Autodesk Inventor part; units mm, degrees
(part 2 of 2)
sketch "Sketch9" plane through (0, 0, 5.08) normal (0, 0, 1) x (1, 0, 0)
  line L0 (165.1, 177.8) -> (175.26, 177.8)
  line L1 (175.26, 177.8) -> (175.26, 172.72)
  line L2 (175.26, 172.72) -> (165.1, 172.72)
  line L3 (165.1, 172.72) -> (165.1, 177.8)
  arc A0 (32.5266, 197.2829) -> (35.5167, 193.04) centre (35.5167, 196.215) ccw projected
  line L4 (32.5266, 197.2829) -> (95.435, 373.4262) projected
  arc A1 (101.6, 372.3583) -> (95.435, 373.4262) centre (98.425, 372.3583) ccw projected
  line L5 (101.6, 372.3583) -> (101.6, 196.215) projected
  arc A2 (98.425, 193.04) -> (101.6, 196.215) centre (98.425, 196.215) ccw projected
  line L6 (98.425, 193.04) -> (35.5167, 193.04) projected
  arc A3 (188.0033, 193.04) -> (190.9934, 197.2829) centre (188.0033, 196.215) ccw projected
  line L7 (188.0033, 193.04) -> (125.095, 193.04) projected
  arc A4 (121.92, 196.215) -> (125.095, 193.04) centre (125.095, 196.215) ccw projected
  line L8 (121.92, 196.215) -> (121.92, 372.3583) projected
  arc A5 (128.085, 373.4262) -> (121.92, 372.3583) centre (125.095, 372.3583) ccw projected
  line L9 (128.085, 373.4262) -> (190.9934, 197.2829) projected
  arc A6 (29.025, 513.5979) -> (22.86, 512.53) centre (26.035, 512.53) ccw projected
  line L10 (29.025, 513.5979) -> (76.0908, 381.8139) projected
  arc A7 (76.0908, 379.6781) -> (76.0908, 381.8139) centre (73.1007, 380.746) ccw projected
  line L11 (76.0908, 379.6781) -> (29.025, 247.8941) projected
  arc A8 (22.86, 248.962) -> (29.025, 247.8941) centre (26.035, 248.962) ccw projected
  line L12 (22.86, 248.962) -> (22.86, 512.53) projected
  line L13 (25.4, 563.88) -> (25.4, 574.04) projected
  line L14 (25.4, 574.04) -> (30.48, 574.04) projected
  line L15 (30.48, 574.04) -> (30.48, 563.88) projected
  line L16 (30.48, 563.88) -> (25.4, 563.88) projected
  line L17 (30.48, 553.72) -> (30.48, 543.56) projected
  line L18 (30.48, 543.56) -> (25.4, 543.56) projected
  line L19 (25.4, 543.56) -> (25.4, 553.72) projected
  line L20 (25.4, 553.72) -> (30.48, 553.72) projected
  line L21 (129.54, 111.578) -> (210.82, 111.578) projected
  line L22 (210.82, 111.578) -> (210.82, 116.84) projected
  line L23 (210.82, 116.84) -> (215.9, 116.84) projected
  line L24 (215.9, 116.84) -> (215.9, 127) projected
  line L25 (215.9, 127) -> (210.82, 127) projected
  line L26 (210.82, 127) -> (210.82, 137.16) projected
  line L27 (210.82, 137.16) -> (215.9, 137.16) projected
  line L28 (215.9, 137.16) -> (215.9, 147.32) projected
  line L29 (215.9, 147.32) -> (210.82, 147.32) projected
  line L30 (210.82, 147.32) -> (210.82, 157.48) projected
  line L31 (210.82, 157.48) -> (215.9, 157.48) projected
  line L32 (215.9, 157.48) -> (215.9, 167.64) projected
  line L33 (215.9, 167.64) -> (210.82, 167.64) projected
  line L34 (210.82, 167.64) -> (210.82, 177.8) projected
  line L35 (210.82, 177.8) -> (215.9, 177.8) projected
  line L36 (215.9, 177.8) -> (215.9, 187.96) projected
  line L37 (215.9, 187.96) -> (76.2, 579.12) projected
  line L38 (76.2, 579.12) -> (0, 579.12) projected
  line L39 (0, 579.12) -> (0, 568.96) projected
  line L40 (0, 568.96) -> (5.08, 568.96) projected
  line L41 (5.08, 568.96) -> (5.08, 558.8) projected
  line L42 (5.08, 558.8) -> (0, 558.8) projected
  line L43 (0, 558.8) -> (0, 548.64) projected
  line L44 (0, 548.64) -> (5.08, 548.64) projected
  line L45 (5.08, 548.64) -> (5.08, 538.48) projected
  line L46 (5.08, 538.48) -> (0, 538.48) projected
  line L47 (0, 538.48) -> (0, 528.32) projected
  line L48 (0, 528.32) -> (5.08, 528.32) projected
  line L49 (5.08, 528.32) -> (5.08, 518.16) projected
  line L50 (5.08, 518.16) -> (0, 518.16) projected
  line L51 (0, 518.16) -> (0, 508) projected
  line L52 (0, 508) -> (5.08, 508) projected
  line L53 (5.08, 508) -> (5.08, 497.84) projected
  line L54 (5.08, 497.84) -> (0, 497.84) projected
  line L55 (0, 497.84) -> (0, 487.68) projected
  line L56 (0, 487.68) -> (5.08, 487.68) projected
  line L57 (5.08, 487.68) -> (5.08, 477.52) projected
  line L58 (5.08, 477.52) -> (0, 477.52) projected
  line L59 (0, 477.52) -> (0, 467.36) projected
  line L60 (0, 467.36) -> (5.08, 467.36) projected
  line L61 (5.08, 467.36) -> (5.08, 457.2) projected
  line L62 (5.08, 457.2) -> (0, 457.2) projected
  line L63 (0, 457.2) -> (0, 447.04) projected
  line L64 (0, 447.04) -> (5.08, 447.04) projected
  line L65 (5.08, 447.04) -> (5.08, 436.88) projected
  line L66 (5.08, 436.88) -> (0, 436.88) projected
  line L67 (0, 436.88) -> (0, 426.72) projected
  line L68 (0, 426.72) -> (5.08, 426.72) projected
  line L69 (5.08, 426.72) -> (5.08, 416.56) projected
  line L70 (5.08, 416.56) -> (0, 416.56) projected
  line L71 (0, 416.56) -> (0, 406.4) projected
  line L72 (0, 406.4) -> (5.08, 406.4) projected
  line L73 (5.08, 406.4) -> (5.08, 396.24) projected
  line L74 (5.08, 396.24) -> (0, 396.24) projected
  line L75 (0, 396.24) -> (0, 386.08) projected
  line L76 (0, 386.08) -> (5.08, 386.08) projected
  line L77 (5.08, 386.08) -> (5.08, 375.92) projected
  line L78 (5.08, 375.92) -> (0, 375.92) projected
  line L79 (0, 375.92) -> (0, 365.76) projected
  line L80 (0, 365.76) -> (5.08, 365.76) projected
  line L81 (5.08, 365.76) -> (5.08, 355.6) projected
  line L82 (5.08, 355.6) -> (0, 355.6) projected
  line L83 (0, 355.6) -> (0, 345.44) projected
  line L84 (0, 345.44) -> (5.08, 345.44) projected
  line L85 (5.08, 345.44) -> (5.08, 335.28) projected
  line L86 (5.08, 335.28) -> (0, 335.28) projected
  line L87 (0, 335.28) -> (0, 325.12) projected
  line L88 (0, 325.12) -> (5.08, 325.12) projected
  line L89 (5.08, 325.12) -> (5.08, 314.96) projected
  line L90 (5.08, 314.96) -> (0, 314.96) projected
  line L91 (0, 314.96) -> (0, 304.8) projected
  line L92 (0, 304.8) -> (5.08, 304.8) projected
  line L93 (5.08, 304.8) -> (5.08, 294.64) projected
  line L94 (5.08, 294.64) -> (0, 294.64) projected
  line L95 (0, 294.64) -> (0, 284.48) projected
  line L96 (0, 284.48) -> (5.08, 284.48) projected
  line L97 (5.08, 284.48) -> (5.08, 274.32) projected
  line L98 (5.08, 274.32) -> (0, 274.32) projected
  line L99 (0, 274.32) -> (0, 264.16) projected
  line L100 (0, 264.16) -> (5.08, 264.16) projected
  line L101 (5.08, 264.16) -> (5.08, 254) projected
  line L102 (5.08, 254) -> (0, 254) projected
  line L103 (0, 254) -> (0, 243.84) projected
  line L104 (0, 243.84) -> (5.08, 243.84) projected
  line L105 (5.08, 243.84) -> (5.08, 233.68) projected
  line L106 (5.08, 233.68) -> (0, 233.68) projected
  line L107 (0, 233.68) -> (0, 223.52) projected
  line L108 (0, 223.52) -> (5.08, 223.52) projected
  line L109 (5.08, 223.52) -> (5.08, 213.36) projected
  line L110 (5.08, 213.36) -> (0, 213.36) projected
  line L111 (0, 213.36) -> (0, 203.2) projected
  line L112 (0, 203.2) -> (5.08, 203.2) projected
  line L113 (5.08, 203.2) -> (5.08, 193.04) projected
  line L114 (5.08, 193.04) -> (0, 193.04) projected
  line L115 (0, 193.04) -> (0, 182.88) projected
  line L116 (0, 182.88) -> (5.08, 182.88) projected
  line L117 (5.08, 182.88) -> (5.08, 172.72) projected
  line L118 (5.08, 172.72) -> (0, 172.72) projected
  line L119 (0, 172.72) -> (0, 162.56) projected
  line L120 (0, 162.56) -> (5.08, 162.56) projected
  line L121 (5.08, 162.56) -> (5.08, 152.4) projected
  line L122 (5.08, 152.4) -> (0, 152.4) projected
  line L123 (0, 152.4) -> (0, 142.24) projected
  line L124 (0, 142.24) -> (5.08, 142.24) projected
  line L125 (5.08, 142.24) -> (5.08, 132.08) projected
  line L126 (5.08, 132.08) -> (0, 132.08) projected
  line L127 (0, 132.08) -> (0, 121.92) projected
  line L128 (0, 121.92) -> (5.08, 121.92) projected
  line L129 (5.08, 121.92) -> (5.08, 111.76) projected
  line L130 (5.08, 111.76) -> (0, 111.76) projected
  line L131 (0, 111.76) -> (0, 111.578) projected
  line L132 (0, 111.578) -> (124.46, 111.578) projected
  line L133 (124.46, 111.578) -> (124.46, 116.84) projected
  line L134 (124.46, 116.84) -> (129.54, 116.84) projected
  line L135 (129.54, 116.84) -> (129.54, 111.578) projected
  line L136 (129.54, 137.16) -> (129.54, 127) projected
  line L137 (129.54, 127) -> (124.46, 127) projected
  line L138 (124.46, 127) -> (124.46, 137.16) projected
  line L139 (124.46, 137.16) -> (129.54, 137.16) projected
  line L140 (129.54, 177.8) -> (129.54, 167.64) projected
  line L141 (129.54, 167.64) -> (124.46, 167.64) projected
  line L142 (124.46, 167.64) -> (124.46, 177.8) projected
  line L143 (124.46, 177.8) -> (129.54, 177.8) projected
  line L144 (129.54, 157.48) -> (129.54, 147.32) projected
  line L145 (129.54, 147.32) -> (124.46, 147.32) projected
  line L146 (124.46, 147.32) -> (124.46, 157.48) projected
  line L147 (124.46, 157.48) -> (129.54, 157.48) projected
  line L148 (144.78, 177.8) -> (154.94, 177.8)
  line L149 (154.94, 177.8) -> (154.94, 172.72)
  line L150 (144.78, 172.72) -> (144.78, 177.8)
  line L151 (154.94, 172.72) -> (144.78, 172.72)
  line L152 (185.42, 177.8) -> (195.58, 177.8)
  line L153 (195.58, 177.8) -> (195.58, 172.72)
  line L154 (185.42, 172.72) -> (185.42, 177.8)
  line L155 (195.58, 172.72) -> (185.42, 172.72)
  line L156 (165.1, 177.8) -> (175.26, 177.8)
  line L157 (175.26, 177.8) -> (175.26, 172.72)
  line L158 (165.1, 172.72) -> (165.1, 177.8)
  line L159 (175.26, 172.72) -> (165.1, 172.72)
  point P0 (0, 0)
  point P1 (170.18, 172.72)
  point P2 (149.86, 172.72)
  point P3 (190.5, 172.72)
  point P4 (170.18, 172.72)
  dimension "d77" = 10.16
  dimension "d78" = 5.08
  dimension "d79" = 81.28
  dimension "d80" = 40.64
  dimension "d81" = 0
  dimension "d84" = 20.32
  dimension "d87" = 20.32
  constraints: 32 end point, 3 horizontal, 2 collinear, 2 parallel, 1 midpoint, 1 perpendicular, 25 other
  measures "d77" distance of L1.end L2.end
  measures "d78" distance of L0.end L1.end
  measures "d79" distance between parallel lines of L34 L140
  measures "d80" distance from line of L140 point (170.18, 172.72)
  measures "d81" distance between parallel lines of L35 L0
  measures "d84" distance of L0.start L148.start
  measures "d87" distance of L0.start L152.start
extrude "Extrusion10" cut sketch "Sketch9" against normal blind 25.4 keep common part
sketch "Sketch10" plane through (0, 0, 5.08) normal (0, 0, 1) x (1, 0, 0)
  line L0 (129.54, 157.48) -> (129.54, 147.32) projected
  line L1 (129.54, 147.32) -> (124.46, 147.32) projected
  line L2 (124.46, 147.32) -> (124.46, 157.48) projected
  line L3 (124.46, 157.48) -> (129.54, 157.48) projected
  line L4 (129.54, 177.8) -> (129.54, 167.64) projected
  line L5 (129.54, 167.64) -> (124.46, 167.64) projected
  line L6 (124.46, 167.64) -> (124.46, 177.8) projected
  line L7 (124.46, 177.8) -> (129.54, 177.8) projected
  line L8 (129.54, 137.16) -> (129.54, 127) projected
  line L9 (129.54, 127) -> (124.46, 127) projected
  line L10 (124.46, 127) -> (124.46, 137.16) projected
  line L11 (124.46, 137.16) -> (129.54, 137.16) projected
  line L12 (129.54, 111.578) -> (210.82, 111.578) projected
  line L13 (210.82, 111.578) -> (210.82, 116.84) projected
  line L14 (210.82, 116.84) -> (215.9, 116.84) projected
  line L15 (215.9, 116.84) -> (215.9, 127) projected
  line L16 (215.9, 127) -> (210.82, 127) projected
  line L17 (210.82, 127) -> (210.82, 137.16) projected
  line L18 (210.82, 137.16) -> (215.9, 137.16) projected
  line L19 (215.9, 137.16) -> (215.9, 147.32) projected
  line L20 (215.9, 147.32) -> (210.82, 147.32) projected
  line L21 (210.82, 147.32) -> (210.82, 157.48) projected
  line L22 (210.82, 157.48) -> (215.9, 157.48) projected
  line L23 (215.9, 157.48) -> (215.9, 167.64) projected
  line L24 (215.9, 167.64) -> (210.82, 167.64) projected
  line L25 (210.82, 167.64) -> (210.82, 177.8) projected
  line L26 (210.82, 177.8) -> (215.9, 177.8) projected
  line L27 (215.9, 177.8) -> (215.9, 187.96) projected
  line L28 (215.9, 187.96) -> (76.2, 579.12) projected
  line L29 (76.2, 579.12) -> (0, 579.12) projected
  line L30 (0, 579.12) -> (0, 568.96) projected
  line L31 (0, 568.96) -> (5.08, 568.96) projected
  line L32 (5.08, 568.96) -> (5.08, 558.8) projected
  line L33 (5.08, 558.8) -> (0, 558.8) projected
  line L34 (0, 558.8) -> (0, 548.64) projected
  line L35 (0, 548.64) -> (5.08, 548.64) projected
  line L36 (5.08, 548.64) -> (5.08, 538.48) projected
  line L37 (5.08, 538.48) -> (0, 538.48) projected
  line L38 (0, 538.48) -> (0, 528.32) projected
  line L39 (0, 528.32) -> (5.08, 528.32) projected
  line L40 (5.08, 528.32) -> (5.08, 518.16) projected
  line L41 (5.08, 518.16) -> (0, 518.16) projected
  line L42 (0, 518.16) -> (0, 508) projected
  line L43 (0, 508) -> (5.08, 508) projected
  line L44 (5.08, 508) -> (5.08, 497.84) projected
  line L45 (5.08, 497.84) -> (0, 497.84) projected
  line L46 (0, 497.84) -> (0, 487.68) projected
  line L47 (0, 487.68) -> (5.08, 487.68) projected
  line L48 (5.08, 487.68) -> (5.08, 477.52) projected
  line L49 (5.08, 477.52) -> (0, 477.52) projected
  line L50 (0, 477.52) -> (0, 467.36) projected
  line L51 (0, 467.36) -> (5.08, 467.36) projected
  line L52 (5.08, 467.36) -> (5.08, 457.2) projected
  line L53 (5.08, 457.2) -> (0, 457.2) projected
  line L54 (0, 457.2) -> (0, 447.04) projected
  line L55 (0, 447.04) -> (5.08, 447.04) projected
  line L56 (5.08, 447.04) -> (5.08, 436.88) projected
  line L57 (5.08, 436.88) -> (0, 436.88) projected
  line L58 (0, 436.88) -> (0, 426.72) projected
  line L59 (0, 426.72) -> (5.08, 426.72) projected
  line L60 (5.08, 426.72) -> (5.08, 416.56) projected
  line L61 (5.08, 416.56) -> (0, 416.56) projected
  line L62 (0, 416.56) -> (0, 406.4) projected
  line L63 (0, 406.4) -> (5.08, 406.4) projected
  line L64 (5.08, 406.4) -> (5.08, 396.24) projected
  line L65 (5.08, 396.24) -> (0, 396.24) projected
  line L66 (0, 396.24) -> (0, 386.08) projected
  line L67 (0, 386.08) -> (5.08, 386.08) projected
  line L68 (5.08, 386.08) -> (5.08, 375.92) projected
  line L69 (5.08, 375.92) -> (0, 375.92) projected
  line L70 (0, 375.92) -> (0, 365.76) projected
  line L71 (0, 365.76) -> (5.08, 365.76) projected
  line L72 (5.08, 365.76) -> (5.08, 355.6) projected
  line L73 (5.08, 355.6) -> (0, 355.6) projected
  line L74 (0, 355.6) -> (0, 345.44) projected
  line L75 (0, 345.44) -> (5.08, 345.44) projected
  line L76 (5.08, 345.44) -> (5.08, 335.28) projected
  line L77 (5.08, 335.28) -> (0, 335.28) projected
  line L78 (0, 335.28) -> (0, 325.12) projected
  line L79 (0, 325.12) -> (5.08, 325.12) projected
  line L80 (5.08, 325.12) -> (5.08, 314.96) projected
  line L81 (5.08, 314.96) -> (0, 314.96) projected
  line L82 (0, 314.96) -> (0, 304.8) projected
  line L83 (0, 304.8) -> (5.08, 304.8) projected
  line L84 (5.08, 304.8) -> (5.08, 294.64) projected
  line L85 (5.08, 294.64) -> (0, 294.64) projected
  line L86 (0, 294.64) -> (0, 284.48) projected
  line L87 (0, 284.48) -> (5.08, 284.48) projected
  line L88 (5.08, 284.48) -> (5.08, 274.32) projected
  line L89 (5.08, 274.32) -> (0, 274.32) projected
  line L90 (0, 274.32) -> (0, 264.16) projected
  line L91 (0, 264.16) -> (5.08, 264.16) projected
  line L92 (5.08, 264.16) -> (5.08, 254) projected
  line L93 (5.08, 254) -> (0, 254) projected
  line L94 (0, 254) -> (0, 243.84) projected
  line L95 (0, 243.84) -> (5.08, 243.84) projected
  line L96 (5.08, 243.84) -> (5.08, 233.68) projected
  line L97 (5.08, 233.68) -> (0, 233.68) projected
  line L98 (0, 233.68) -> (0, 223.52) projected
  line L99 (0, 223.52) -> (5.08, 223.52) projected
  line L100 (5.08, 223.52) -> (5.08, 213.36) projected
  line L101 (5.08, 213.36) -> (0, 213.36) projected
  line L102 (0, 213.36) -> (0, 203.2) projected
  line L103 (0, 203.2) -> (5.08, 203.2) projected
  line L104 (5.08, 203.2) -> (5.08, 193.04) projected
  line L105 (5.08, 193.04) -> (0, 193.04) projected
  line L106 (0, 193.04) -> (0, 182.88) projected
  line L107 (0, 182.88) -> (5.08, 182.88) projected
  line L108 (5.08, 182.88) -> (5.08, 172.72) projected
  line L109 (5.08, 172.72) -> (0, 172.72) projected
  line L110 (0, 172.72) -> (0, 162.56) projected
  line L111 (0, 162.56) -> (5.08, 162.56) projected
  line L112 (5.08, 162.56) -> (5.08, 152.4) projected
  line L113 (5.08, 152.4) -> (0, 152.4) projected
  line L114 (0, 152.4) -> (0, 142.24) projected
  line L115 (0, 142.24) -> (5.08, 142.24) projected
  line L116 (5.08, 142.24) -> (5.08, 132.08) projected
  line L117 (5.08, 132.08) -> (0, 132.08) projected
  line L118 (0, 132.08) -> (0, 121.92) projected
  line L119 (0, 121.92) -> (5.08, 121.92) projected
  line L120 (5.08, 121.92) -> (5.08, 111.76) projected
  line L121 (5.08, 111.76) -> (0, 111.76) projected
  line L122 (0, 111.76) -> (0, 111.578) projected
  line L123 (0, 111.578) -> (124.46, 111.578) projected
  line L124 (124.46, 111.578) -> (124.46, 116.84) projected
  line L125 (124.46, 116.84) -> (129.54, 116.84) projected
  line L126 (129.54, 116.84) -> (129.54, 111.578) projected
  line L127 (30.48, 553.72) -> (30.48, 543.56) projected
  line L128 (30.48, 543.56) -> (25.4, 543.56) projected
  line L129 (25.4, 543.56) -> (25.4, 553.72) projected
  line L130 (25.4, 553.72) -> (30.48, 553.72) projected
  line L131 (25.4, 563.88) -> (25.4, 574.04) projected
  line L132 (25.4, 574.04) -> (30.48, 574.04) projected
  line L133 (30.48, 574.04) -> (30.48, 563.88) projected
  line L134 (30.48, 563.88) -> (25.4, 563.88) projected
  arc A0 (29.025, 513.5979) -> (22.86, 512.53) centre (26.035, 512.53) ccw projected
  line L135 (29.025, 513.5979) -> (76.0908, 381.8139) projected
  arc A1 (76.0908, 379.6781) -> (76.0908, 381.8139) centre (73.1007, 380.746) ccw projected
  line L136 (76.0908, 379.6781) -> (29.025, 247.8941) projected
  arc A2 (22.86, 248.962) -> (29.025, 247.8941) centre (26.035, 248.962) ccw projected
  line L137 (22.86, 248.962) -> (22.86, 512.53) projected
  arc A3 (188.0033, 193.04) -> (190.9934, 197.2829) centre (188.0033, 196.215) ccw projected
  line L138 (188.0033, 193.04) -> (125.095, 193.04) projected
  arc A4 (121.92, 196.215) -> (125.095, 193.04) centre (125.095, 196.215) ccw projected
  line L139 (121.92, 196.215) -> (121.92, 372.3583) projected
  arc A5 (128.085, 373.4262) -> (121.92, 372.3583) centre (125.095, 372.3583) ccw projected
  line L140 (128.085, 373.4262) -> (190.9934, 197.2829) projected
  arc A6 (32.5266, 197.2829) -> (35.5167, 193.04) centre (35.5167, 196.215) ccw projected
  line L141 (32.5266, 197.2829) -> (95.435, 373.4262) projected
  arc A7 (101.6, 372.3583) -> (95.435, 373.4262) centre (98.425, 372.3583) ccw projected
  line L142 (101.6, 372.3583) -> (101.6, 196.215) projected
  arc A8 (98.425, 193.04) -> (101.6, 196.215) centre (98.425, 196.215) ccw projected
  line L143 (98.425, 193.04) -> (35.5167, 193.04) projected
  line L144 (165.1, 177.8) -> (165.1, 172.72) projected
  line L145 (175.26, 177.8) -> (165.1, 177.8) projected
  line L146 (175.26, 172.72) -> (175.26, 177.8) projected
  line L147 (165.1, 172.72) -> (175.26, 172.72) projected
  line L148 (144.78, 177.8) -> (144.78, 172.72) projected
  line L149 (154.94, 177.8) -> (144.78, 177.8) projected
  line L150 (154.94, 172.72) -> (154.94, 177.8) projected
  line L151 (144.78, 172.72) -> (154.94, 172.72) projected
  line L152 (185.42, 177.8) -> (185.42, 172.72) projected
  line L153 (195.58, 177.8) -> (185.42, 177.8) projected
  line L154 (195.58, 172.72) -> (195.58, 177.8) projected
  line L155 (185.42, 172.72) -> (195.58, 172.72) projected
  line L156 (50.8, 579.12) -> (50.8, 513.0437)
  line L157 (50.8, 513.0437) -> (92.6537, 395.8533)
  line L158 (92.6537, 395.8533) -> (141.6524, 395.8533)
  line L159 (50.8, 579.12) -> (68.5955, 616.8382)
  line L160 (68.5955, 616.8382) -> (148.9717, 515.6585)
  line L161 (148.9717, 515.6585) -> (141.6524, 395.8533)
  line L162 (76.2, 579.12) -> (215.9, 187.96) projected
  line L163 (29.025, 513.5979) -> (76.0908, 381.8139) projected
  arc A9 (128.085, 373.4262) -> (121.92, 372.3583) centre (125.095, 372.3583) ccw construction
  line L164 (83.9426, 375.5333) -> (124.46, 375.5333) construction
  arc A10 (101.6, 372.3583) -> (95.435, 373.4262) centre (98.425, 372.3583) ccw construction
  point P0 (0, 0)
  point P1 (117.153, 395.8533)
  dimension "d92" = 20.32
  dimension "d93" = 20.32
  dimension "d94" = 20.32
  dimension "d95" = 20.32
  constraints: 14 end point, 4 point on line, 2 horizontal, 1 midpoint, 1 parallel, 1 tangent, 1 vertical
  measures "d92" distance between parallel lines of L156 L127
  measures "d93" distance between parallel lines of L141 L136
  measures "d94" distance between parallel lines of L135 L157
  measures "d95" distance between parallel lines of L164 L158
extrude "Extrusion11" cut sketch "Sketch10" against normal blind 25.4 contours L158 L157 L156 L29 L28 | L28 L29 L159 L160 L161
chamfer "Chamfer1" distance 12.7 angle 45 1 edges at (50.8, 579.12, 2.54)
sketch "Sketch11" plane through (0, 0, 5.08) normal (0, 0, 1) x (1, 0, 0)
  point P0 (0, 0)
equation "\"d4\" = d3"
equation "\"d7\" = 2 * d3"
equation "\"d22\" = d21"
equation "\"d29\" = d27"
equation "\"d62\" = d61"
equation "\"d63\" = d61"
equation "\"d64\" = d61"
equation "\"d65\" = d64"
equation "\"d66\" = d65"
equation "\"d69\" = 0.5 * d101"
equation "\"d72\" = 2 * d69"
equation "\"d80\" = 0.5 * d79"
equation "\"d92\" = d94"
equation "\"d94\" = d93"
equation "\"d95\" = d94"
body "Solid2"
